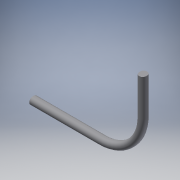
# Autodesk Inventor part: pipe2
Saved by Autodesk Inventor 2019 (Build 230136000, 136)
## iProperties
Created: 2019-11-19
Part Number: pipe2
Material: Generic
Document SubType Name: Modeling
Designer: Administrator
Density: 1 g/cm^3
Appearance: Default
Author: Administrator
Autodesk Inventor part; units mm, degrees
ref_plane "YZ Plane" through (0, 0, 0) normal (1, 0, 0) x (0, 1, 0)
ref_plane "XZ Plane" through (0, 0, 0) normal (0, 1, 0) x (-1, 0, 0)
ref_plane "XY Plane" through (0, 0, 0) normal (0, 0, 1) x (1, 0, 0)
sketch "Sketch1" plane through (0, 0, 0) normal (0, 0, 1) x (1, 0, 0)
  line L0 (0, 0) -> (95.9616, 0)
  line L1 (0, 0) -> (0, 9.8571)
  line L2 (0, 9.8571) -> (78.8567, 9.8571)
  arc A0 (95.9616, 0) -> (157.7134, 61.7524) centre (95.9616, 61.7517) ccw
  line L3 (78.8567, 9.8571) -> (95.9616, 9.8571)
  arc A1 (95.9616, 9.8571) -> (147.8563, 61.7517) centre (95.9616, 61.7517) ccw
  line L4 (147.8563, 61.7517) -> (147.8563, 112.8865)
  line L5 (147.8563, 112.8865) -> (157.7134, 112.8865)
  line L6 (157.7134, 112.8865) -> (157.7134, 61.7524)
  constraints: 14 end point, 4 point on circle, 3 perpendicular, 2 centre point, 2 horizontal, 2 tangent, 2 vertical, 1 concentric
extrude "Extrusion1" add sketch "Sketch1" along normal blind 11.1125
fillet "Fillet1" radius 4.7625 12 edges at (132.6567, 25.0567, 0) (147.8563, 87.3191, 0) (39.4283, 9.8571, 0) (132.6567, 25.0567, 11.1125) (147.8563, 87.3191, 11.1125) (39.4283, 9.8571, 11.1125) (139.6269, 18.0869, 11.1125) (157.7134, 87.3194, 11.1125) (47.9808, 0, 11.1125) (157.7134, 87.3194, 0) (47.9808, 0, 0) (139.6269, 18.0869, 0)
shell "Shell1" thickness 2.667 removed faces 1 at (152.8402, 112.8865, 3.175)
body "Solid1"
